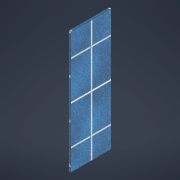
# Autodesk Inventor part: SolarPanel
Saved by Autodesk Inventor 2022 (Build 260153000, 153)
## iProperties
Created: 2022-07-14
Part Number: SolarPanel
Material: Glass
Document SubType Name: Modeling
Designer: ForseFire
Density: 2.18 g/cm^3
Appearance: 1.5in Square - Medium Blue
Author: ForseFire
Autodesk Inventor part; units mm, degrees
ref_plane "YZ Plane" through (0, 0, 0) normal (1, 0, 0) x (0, 1, 0)
ref_plane "XZ Plane" through (0, 0, 0) normal (0, 1, 0) x (-1, 0, 0)
ref_plane "XY Plane" through (0, 0, 0) normal (0, 0, 1) x (1, 0, 0)
sketch "Sketch1" plane through (0, 0, 0) normal (1, 0, 0) x (0, 1, 0)
  line L0 (-60, -20) -> (60, -20)
  line L1 (60, -20) -> (60, 20)
  line L2 (60, 20) -> (-60, 20)
  line L3 (-60, 20) -> (-60, -20)
  line L4 (-60, -20) -> (60, 20) construction
  line L5 (60, -20) -> (-60, 20) construction
  point P0 (0, 0)
  dimension "d0" = 120
  dimension "d1" = 40
  constraints: 12 end point, 2 midpoint, 2 parallel, 1 horizontal, 1 perpendicular
  measures "d0" distance of L2.end L1.end
  measures "d1" distance of L1.end L0.end
extrude "Extrusion1" add sketch "Sketch1" along normal blind 2
body "Solid1"
